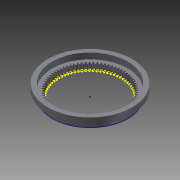
# Autodesk Inventor part: Stirnzahnrad1
Saved by Autodesk Inventor 2014 (Build 180170000, 170)
## iProperties
Created: 2013-05-23
Part Number: Stirnzahnrad1
Material: Steel
Document SubType Name: Modeling
Designer: hartmann
Categories: <?xml version="1.0" encoding="UTF-16"?> <MemberInstance><Categories><FamilyTemplate><FamilyTemplateParameter ValueType="xs:double" Id="1" ObjectReferenceKey="da_z" ObjectType="kUserParameterObject"/><FamilyTemplateParameter ValueType="xs:double" Id="2" ObjectReferenceKey="da_b" ObjectType="kUserParameterObject"/><FamilyTemplateParameter ValueType="xs:double" Id="3" ObjectReferenceKey="da_beta" ObjectType="kUserParameterObject"/><FamilyTemplateParameter ValueType="xs:double" Id="4" ObjectReferenceKey="da_da" ObjectType="kUserParameterObject"/><FamilyTemplateParameter ValueType="xs:double" Id="5" ObjectReferenceKey="da_aw" ObjectType="kUserParameterObject"/><FamilyTemplateParameter ValueType="xs:string" Id="6" ObjectReferenceKey="EAIAABAAAACIAQAAAAAAAIAAAAAAAAAA" ObjectType="83910656" SubObjectId="SurfaceGeometry"/></FamilyTemplate><ParamToTemplateMap><ParamToTemplate CategoryParameter="//CategoryParameter[@InternalName='046C89C9-8512-4d59-83FE-43B91F4F132A']" TemplateParameter="1"/><ParamToTemplate CategoryParameter="//CategoryParameter[@InternalName='2552DF32-E462-4b46-AEBF-C6C7768E72AC']" TemplateParameter="2"/><ParamToTemplate CategoryParameter="//CategoryParameter[@InternalName='C9EE641D-15FC-4fae-A226-E94C4372FDD7']" TemplateParameter="3"/><ParamToTemplate><ParamToTemplate CategoryParameter="//CategoryParameter[@InternalName='00B6519A-459B-49c7-AD84-2E56D39A5744']" ConstantValue="0.000000"/></ParamToTemplate><ParamToTemplate><ParamToTemplate CategoryParameter="//CategoryParameter[@InternalName='04B31F0E-C7A6-4894-AA32-9629BEFACF47']" ConstantValue="1.000000"/></ParamToTemplate><ParamToTemplate><ParamToTemplate CategoryParameter="//CategoryParameter[@InternalName='43CBEC2E-7847-49e7-A936-2F7889FCB2D9']" ConstantValue="0.250000"/></ParamToTemplate><ParamToTemplate><ParamToTemplate CategoryParameter="//CategoryParameter[@InternalName='B1EFC894-105D-4ebd-86BF-FA20ED196853']" ConstantValue="0.350000"/></ParamToTemplate><ParamToTemplate><ParamToTemplate CategoryParameter="//CategoryParameter[@InternalName='51175063-3D10-4879-93E8-6246FE8B403D']" ConstantValue="2060000000.000000"/></ParamToTemplate><ParamToTemplate><ParamToTemplate CategoryParameter="//CategoryParameter[@InternalName='A3A52E27-4454-46a9-B0BD-C932399B70AF']" ConstantValue="0.300000"/></ParamToTemplate><ParamToTemplate><ParamToTemplate CategoryParameter="//CategoryParameter[@InternalName='91B76062-C214-41d9-B1B9-14D2AB99603D']" ConstantValue="0.030000"/></ParamToTemplate><ParamToTemplate><ParamToTemplate CategoryParameter="//CategoryParameter[@InternalName='374E806E-8B8A-4dda-A9AA-1039D6500AD2']" ConstantValue="33.333333"/></ParamToTemplate><ParamToTemplate><ParamToTemplate CategoryParameter="//CategoryParameter[@InternalName='2D373A89-B862-43d6-8D0B-0CBF12AB9F6C']" ConstantValue="0.349066"/></ParamToTemplate><ParamToTemplate CategoryParameter="//CategoryParameter[@InternalName='37777632-D6A2-4fac-9D53-DB8ACD95C989']" TemplateParameter="4"/><ParamToTemplate CategoryParameter="//CategoryParameter[@InternalName='FD1017F1-B727-4f7e-9707-0F86F1FF9423']" TemplateParameter="5"/><ParamToTemplate><ParamToTemplate CategoryParameter="//CategoryParameter[@InternalName='9E1B4470-B2D3-4ff1-B813-535BB4CDF51A']" ConstantValue="3520000.000000"/></ParamToTemplate><ParamToTemplate><ParamToTemplate CategoryParameter="//CategoryParameter[@InternalName='F8452263-BFF6-458c-9FB1-07C4B99E95CD']" ConstantValue="11400000.000000"/></ParamToTemplate><ParamToTemplate><ParamToTemplate CategoryParameter="//CategoryParameter[@InternalName='3E3BB259-FD49-497f-8171-6EBC954A3479']" ConstantValue="2.000000"/></ParamToTemplate><ParamToTemplate CategoryParameter="//CategoryParameter[@InternalName='27C3BAF2-7550-4e4b-AE2C-0DB134B7D9B7']" TemplateParameter="6"/></ParamToTemplateMap><Category DisplayName="Gear" InternalName="DC85795E-93AB-48d5-8EEE-5A27447B64BD" Mnemonic="Gear"><CategoryParameter DisplayName="z" InternalName="046C89C9-8512-4d59-83FE-43B91F4F132A" Mnemonic="z"/><CategoryParameter DisplayName="b" InternalName="2552DF32-E462-4b46-AEBF-C6C7768E72AC" Mnemonic="b"/><CategoryParameter DisplayName="||b|" InternalName="C9EE641D-15FC-4fae-A226-E94C4372FDD7" Mnemonic="beta"/><CategoryParameter DisplayName="x" InternalName="00B6519A-459B-49c7-AD84-2E56D39A5744" Mnemonic="x"/><CategoryParameter DisplayName="a*" InternalName="04B31F0E-C7A6-4894-AA32-9629BEFACF47" Mnemonic="a"/><CategoryParameter DisplayName="c*" InternalName="43CBEC2E-7847-49e7-A936-2F7889FCB2D9" Mnemonic="c"/><CategoryParameter DisplayName="r|.f|*" InternalName="B1EFC894-105D-4ebd-86BF-FA20ED196853" Mnemonic="rf"/><CategoryParameter DisplayName="E" InternalName="51175063-3D10-4879-93E8-6246FE8B403D" Mnemonic="E"/><CategoryParameter DisplayName="||m|" InternalName="A3A52E27-4454-46a9-B0BD-C932399B70AF" Mnemonic="mi"/><Category DisplayName="SpurGear" InternalName="26C5A22E-A91E-4dfd-A3B3-23CCAFAE1764" Mnemonic="SpurGear"><CategoryParameter DisplayName="m" InternalName="91B76062-C214-41d9-B1B9-14D2AB99603D" Mnemonic="m"/><CategoryParameter DisplayName="P" InternalName="374E806E-8B8A-4dda-A9AA-1039D6500AD2" Mnemonic="PP"/><CategoryParameter DisplayName="||a|" InternalName="2D373A89-B862-43d6-8D0B-0CBF12AB9F6C" Mnemonic="alpha"/><CategoryParameter DisplayName="d|.a|" InternalName="37777632-D6A2-4fac-9D53-DB8ACD95C989" Mnemonic="da"/><CategoryParameter DisplayName="a|.w|" InternalName="FD1017F1-B727-4f7e-9707-0F86F1FF9423" Mnemonic="aw"/><CategoryParameter DisplayName="||s||.Flim|" InternalName="9E1B4470-B2D3-4ff1-B813-535BB4CDF51A" Mnemonic="sFlim"/><CategoryParameter DisplayName="||s||.Hlim|" InternalName="F8452263-BFF6-458c-9FB1-07C4B99E95CD" Mnemonic="sHlim"/><CategoryParameter DisplayName="Typ" InternalName="3E3BB259-FD49-497f-8171-6EBC954A3479" Mnemonic="type"/><Category DisplayName="InternalSpurGear" InternalName="7CF704F6-14A9-42f8-93CE-E71DF57C2B55" Mnemonic="InternalSpurGear"><CategoryParameter DisplayName="PitchDiameter" InternalName="27C3BAF2-7550-4e4b-AE2C-0DB134B7D9B7" Mnemonic="IDS_PITCHDIAM"/></Category></Category></Category></Categories></MemberInstance>
Density: 1 g/cm^3
Appearance: Steel
CustomPartVersion: 1
Author: hartmann
Autodesk Inventor part; units mm, degrees
sketch "Sketch1" plane through (0, 0, 0) normal (0, 0, 1) x (1, 0, 0)
  circle A0 centre (0, 0) radius 12.7875
  dimension "d0" = 25.575
  constraints: 1 centre point
  measures "d0" diameter of A0
extrude "Extrusion1" add sketch "Sketch1" along normal blind 2
ref_plane "Work Plane2" through (0, 0, 1) normal (0, 0, 1) x (1, 0, 0)
sketch "Sketch2" plane through (0, 0, 0) normal (0, 0, -1) x (-1, 0, 0)
  circle A0 centre (0, 0) radius 12.7875 projected
  circle A1 centre (0, 0) radius 11.25
  dimension "d3" = 22.5
  constraints: 1 centre point, 1 coincident
  measures "d3" diameter of A1
surface extrude "Flankendurchmesser" sketch "Sketch2" against normal through all shown no curves A1
ref_plane "Work Plane8" through (0, 0, 0) normal (0.9991228, 0.0418757, 0) x (0, 0, 1)
ref_plane "Work Plane9" through (0, 0, 0) normal (1, 0, 0) x (0, 1, 0)
spur gear teeth "Stirnzahnrad" teeth 75 pitch diameter 22.5 tip diameter 21.9 root diameter 23.25 face width 2 start plane through (0, 0, 0) normal (0, 0, -1) x (-1, 0, 0)
sketch "Skizze4" plane through (0, 0, 2) normal (0, 0, 1) x (1, 0, 0)
  circle A0 centre (0, 0) radius 12.7875 projected
  circle A1 centre (0, 0) radius 14.2875
  arc A2 (1.2586, -10.8774) -> (1.4861, -10.8487) centre (0, 0) ccw projected
  circle A3 centre (0, 0) radius 14.2875
  dimension "d53" = 1.5
  constraints: 2 centre point, 2 coincident, 1 concentric
  measures "d53" radial gap between concentric circles of A0 A1
extrude "Extrusion2" add sketch "Skizze4" along normal blind 2
sketch "Skizze6" plane through (0, 0, 0) normal (0, 0, -1) x (-1, 0, 0)
  arc A0 (-1.2586, -10.8774) -> (-1.094, -11.5734) centre (2.6832, -10.3129) ccw projected
  arc A1 (-1.4861, -10.8487) -> (-1.2586, -10.8774) centre (0, 0) ccw projected
  arc A2 (-1.8186, -11.4819) -> (-1.4861, -10.8487) centre (-5.1636, -9.3216) ccw projected
  arc A3 (-2.0586, -11.4413) -> (-1.8186, -11.4819) centre (0, 0) ccw projected
  arc A4 (-2.1643, -10.734) -> (-2.0586, -11.4413) centre (1.8108, -10.5013) ccw projected
  arc A5 (-2.3887, -10.6863) -> (-2.1643, -10.734) centre (0, 0) ccw projected
  arc A6 (-2.773, -11.2894) -> (-2.3887, -10.6863) centre (-5.9255, -8.8569) ccw projected
  arc A7 (-3.0088, -11.2289) -> (-2.773, -11.2894) centre (0, 0) ccw projected
  arc A8 (-3.055, -10.5152) -> (-3.0088, -11.2289) centre (0.9257, -10.616) ccw projected
  arc A9 (-3.2745, -10.4489) -> (-3.055, -10.5152) centre (0, 0) ccw projected
  arc A10 (-3.7079, -11.0178) -> (-3.2745, -10.4489) centre (-6.6458, -8.33) ccw projected
  arc A11 (-3.9378, -10.9377) -> (-3.7079, -11.0178) centre (0, 0) ccw projected
  arc A12 (-3.9241, -10.2227) -> (-3.9378, -10.9377) centre (0.0342, -10.6562) ccw projected
  arc A13 (-4.1374, -10.1383) -> (-3.9241, -10.2227) centre (0, 0) ccw projected
  arc A14 (-4.6168, -10.6689) -> (-4.1374, -10.1383) centre (-7.3196, -7.7446) ccw projected
  arc A15 (-4.8393, -10.5699) -> (-4.6168, -10.6689) centre (0, 0) ccw projected
  arc A16 (-4.7658, -9.8585) -> (-4.8393, -10.5699) centre (-0.8576, -10.6217) ccw projected
  arc A17 (-4.9712, -9.7565) -> (-4.7658, -9.8585) centre (0, 0) ccw projected
  arc A18 (-5.4934, -10.2452) -> (-4.9712, -9.7565) centre (-7.942, -7.105) ccw projected
  arc A19 (-5.7068, -10.1279) -> (-5.4934, -10.2452) centre (0, 0) ccw projected
  arc A20 (-5.574, -9.4251) -> (-5.7068, -10.1279) centre (-1.7434, -10.5127) ccw projected
  arc A21 (-5.7702, -9.3063) -> (-5.574, -9.4251) centre (0, 0) ccw projected
  arc A22 (-6.3314, -9.7495) -> (-5.7702, -9.3063) centre (-8.5086, -6.4155) ccw projected
  arc A23 (-6.5342, -9.6148) -> (-6.3314, -9.7495) centre (0, 0) ccw projected
  arc A24 (-6.3431, -8.9256) -> (-6.5342, -9.6148) centre (-2.617, -10.3299) ccw projected
  arc A25 (-6.5287, -8.7909) -> (-6.3431, -8.9256) centre (0, 0) ccw projected
  arc A26 (-7.125, -9.1856) -> (-6.5287, -8.7909) centre (-9.0156, -5.681) ccw projected
  arc A27 (-7.3158, -9.0343) -> (-7.125, -9.1856) centre (0, 0) ccw projected
  arc A28 (-7.0678, -8.3636) -> (-7.3158, -9.0343) centre (-3.4722, -10.0747) ccw projected
  arc A29 (-7.2414, -8.2137) -> (-7.0678, -8.3636) centre (0, 0) ccw projected
  arc A30 (-7.8687, -8.5571) -> (-7.2414, -8.2137) centre (-9.4594, -4.9067) ccw projected
  arc A31 (-8.0462, -8.3905) -> (-7.8687, -8.5571) centre (0, 0) ccw projected
  arc A32 (-7.7428, -7.7428) -> (-8.0462, -8.3905) centre (-4.3031, -9.7488) ccw projected
  arc A33 (-7.9033, -7.579) -> (-7.7428, -7.7428) centre (0, 0) ccw projected
  arc A34 (-8.5571, -7.8687) -> (-7.9033, -7.579) centre (-9.8368, -4.0979) ccw projected
  arc A35 (-8.72, -7.6878) -> (-8.5571, -7.8687) centre (0, 0) ccw projected
  arc A36 (-8.3636, -7.0678) -> (-8.72, -7.6878) centre (-5.1037, -9.3545) ccw projected
  arc A37 (-8.5097, -6.8911) -> (-8.3636, -7.0678) centre (0, 0) ccw projected
  arc A38 (-9.1856, -7.125) -> (-8.5097, -6.8911) centre (-10.1452, -3.2605) ccw projected
  arc A39 (-9.3328, -6.9311) -> (-9.1856, -7.125) centre (0, 0) ccw projected
  arc A40 (-8.9256, -6.3431) -> (-9.3328, -6.9311) centre (-5.8686, -8.8947) ccw projected
  arc A41 (-9.0565, -6.1548) -> (-8.9256, -6.3431) centre (0, 0) ccw projected
  arc A42 (-9.7495, -6.3314) -> (-9.0565, -6.1548) centre (-10.3824, -2.4001) ccw projected
  arc A43 (-9.88, -6.1259) -> (-9.7495, -6.3314) centre (0, 0) ccw projected
  arc A44 (-9.4251, -5.574) -> (-9.88, -6.1259) centre (-6.5923, -8.3724) ccw projected
  arc A45 (-9.5398, -5.3754) -> (-9.4251, -5.574) centre (0, 0) ccw projected
  arc A46 (-10.2452, -5.4934) -> (-9.5398, -5.3754) centre (-10.5469, -1.5229) ccw projected
  arc A47 (-10.358, -5.2776) -> (-10.2452, -5.4934) centre (0, 0) ccw projected
  arc A48 (-9.8585, -4.7658) -> (-10.358, -5.2776) centre (-7.2698, -7.7914) ccw projected
  arc A49 (-9.9561, -4.5583) -> (-9.8585, -4.7658) centre (0, 0) ccw projected
  arc A50 (-10.6689, -4.6168) -> (-9.9561, -4.5583) centre (-10.6373, -0.635) ccw projected
  arc A51 (-10.7632, -4.3924) -> (-10.6689, -4.6168) centre (0, 0) ccw projected
  arc A52 (-10.2227, -3.9241) -> (-10.7632, -4.3924) centre (-7.8962, -7.1558) ccw projected
  arc A53 (-10.3026, -3.7092) -> (-10.2227, -3.9241) centre (0, 0) ccw projected
  arc A54 (-11.0178, -3.7079) -> (-10.3026, -3.7092) centre (-10.6531, 0.2573) ccw projected
  arc A55 (-11.093, -3.4763) -> (-11.0178, -3.7079) centre (0, 0) ccw projected
  arc A56 (-10.5152, -3.055) -> (-11.093, -3.4763) centre (-8.4673, -6.4699) ccw projected
  arc A57 (-10.5769, -2.8341) -> (-10.5152, -3.055) centre (0, 0) ccw projected
  arc A58 (-11.2894, -2.773) -> (-10.5769, -2.8341) centre (-10.5942, 1.1479) ccw projected
  arc A59 (-11.345, -2.5359) -> (-11.2894, -2.773) centre (0, 0) ccw projected
  arc A60 (-10.734, -2.1643) -> (-11.345, -2.5359) centre (-8.979, -5.7387) ccw projected
  arc A61 (-10.7769, -1.9391) -> (-10.734, -2.1643) centre (0, 0) ccw projected
  arc A62 (-11.4819, -1.8186) -> (-10.7769, -1.9391) centre (-10.461, 2.0303) ccw projected
  arc A63 (-11.5174, -1.5777) -> (-11.4819, -1.8186) centre (0, 0) ccw projected
  arc A64 (-10.8774, -1.2586) -> (-11.5174, -1.5777) centre (-9.4277, -4.9672) ccw projected
  arc A65 (-10.9014, -1.0305) -> (-10.8774, -1.2586) centre (0, 0) ccw projected
  arc A66 (-11.5938, -0.8514) -> (-10.9014, -1.0305) centre (-10.2545, 2.8986) ccw projected
  arc A67 (-11.6091, -0.6084) -> (-11.5938, -0.8514) centre (0, 0) ccw projected
  arc A68 (-10.9446, -0.3439) -> (-11.6091, -0.6084) centre (-9.8103, -4.1609) ccw projected
  arc A69 (-10.9494, -0.1147) -> (-10.9446, -0.3439) centre (0, 0) ccw projected
  arc A70 (-11.6244, 0.1217) -> (-10.9494, -0.1147) centre (-9.9759, 3.7465) ccw projected
  arc A71 (-11.6193, 0.3652) -> (-11.6244, 0.1217) centre (0, 0) ccw projected
  arc A72 (-10.935, 0.5731) -> (-11.6193, 0.3652) centre (-10.1241, -3.3254) ccw projected
  arc A73 (-10.9206, 0.802) -> (-10.935, 0.5731) centre (0, 0) ccw projected
  arc A74 (-11.5734, 1.094) -> (-10.9206, 0.802) centre (-9.6275, 4.5681) ccw projected
  arc A75 (-11.548, 1.3361) -> (-11.5734, 1.094) centre (0, 0) ccw projected
  arc A76 (-10.8487, 1.4861) -> (-11.548, 1.3361) centre (-10.3668, -2.4666) ccw projected
  arc A77 (-10.8152, 1.713) -> (-10.8487, 1.4861) centre (0, 0) ccw projected
  arc A78 (-11.4413, 2.0586) -> (-10.8152, 1.713) centre (-9.2114, 5.3577) ccw projected
  arc A79 (-11.3957, 2.2978) -> (-11.4413, 2.0586) centre (0, 0) ccw projected
  arc A80 (-10.6863, 2.3887) -> (-11.3957, 2.2978) centre (-10.5369, -1.5905) ccw projected
  arc A81 (-10.6339, 2.6119) -> (-10.6863, 2.3887) centre (0, 0) ccw projected
  arc A82 (-11.2289, 3.0088) -> (-10.6339, 2.6119) centre (-8.7308, 6.1097) ccw projected
  arc A83 (-11.1634, 3.2433) -> (-11.2289, 3.0088) centre (0, 0) ccw projected
  arc A84 (-10.4489, 3.2745) -> (-11.1634, 3.2433) centre (-10.633, -0.7032) ccw projected
  arc A85 (-10.3781, 3.4926) -> (-10.4489, 3.2745) centre (0, 0) ccw projected
  arc A86 (-10.9377, 3.9378) -> (-10.3781, 3.4926) centre (-8.189, 6.8188) ccw projected
  arc A87 (-10.8529, 4.166) -> (-10.9377, 3.9378) centre (0, 0) ccw projected
  arc A88 (-10.1383, 4.1374) -> (-10.8529, 4.166) centre (-10.6546, 0.189) ccw projected
  arc A89 (-10.0494, 4.3488) -> (-10.1383, 4.1374) centre (0, 0) ccw projected
  arc A90 (-10.5699, 4.8393) -> (-10.0494, 4.3488) centre (-7.5897, 7.4802) ccw projected
  arc A91 (-10.4662, 5.0596) -> (-10.5699, 4.8393) centre (0, 0) ccw projected
  arc A92 (-9.7565, 4.9712) -> (-10.4662, 5.0596) centre (-10.6014, 1.0799) ccw projected
  arc A93 (-9.6503, 5.1744) -> (-9.7565, 4.9712) centre (0, 0) ccw projected
  arc A94 (-10.1279, 5.7068) -> (-9.6503, 5.1744) centre (-6.9371, 8.089) ccw projected
  arc A95 (-10.0061, 5.9176) -> (-10.1279, 5.7068) centre (0, 0) ccw projected
  arc A96 (-9.3063, 5.7702) -> (-10.0061, 5.9176) centre (-10.4738, 1.9632) ccw projected
  arc A97 (-9.1834, 5.9638) -> (-9.3063, 5.7702) centre (0, 0) ccw projected
  arc A98 (-9.6148, 6.5342) -> (-9.1834, 5.9638) centre (-6.2359, 8.6411) ccw projected
  arc A99 (-9.4759, 6.7341) -> (-9.6148, 6.5342) centre (0, 0) ccw projected
  arc A100 (-8.7909, 6.5287) -> (-9.4759, 6.7341) centre (-10.2728, 2.8328) ccw projected
  arc A101 (-8.6522, 6.7113) -> (-8.7909, 6.5287) centre (0, 0) ccw projected
  arc A102 (-9.0343, 7.3158) -> (-8.6522, 6.7113) centre (-5.491, 9.1326) ccw projected
  arc A103 (-8.8791, 7.5034) -> (-9.0343, 7.3158) centre (0, 0) ccw projected
  arc A104 (-8.2137, 7.2414) -> (-8.8791, 7.5034) centre (-9.9998, 3.6824) ccw projected
  arc A105 (-8.0603, 7.4118) -> (-8.2137, 7.2414) centre (0, 0) ccw projected
  arc A106 (-8.3905, 8.0462) -> (-8.0603, 7.4118) centre (-4.7075, 9.5601) ccw projected
  arc A107 (-8.2201, 8.2201) -> (-8.3905, 8.0462) centre (0, 0) ccw projected
  arc A108 (-7.579, 7.9033) -> (-8.2201, 8.2201) centre (-9.6566, 4.5063) ccw projected
  arc A109 (-7.4118, 8.0603) -> (-7.579, 7.9033) centre (0, 0) ccw projected
  arc A110 (-7.6878, 8.72) -> (-7.4118, 8.0603) centre (-3.891, 9.9205) ccw projected
  arc A111 (-7.5034, 8.8791) -> (-7.6878, 8.72) centre (0, 0) ccw projected
  arc A112 (-6.8911, 8.5097) -> (-7.5034, 8.8791) centre (-9.2456, 5.2985) ccw projected
  arc A113 (-6.7113, 8.6522) -> (-6.8911, 8.5097) centre (0, 0) ccw projected
  arc A114 (-6.9311, 9.3328) -> (-6.7113, 8.6522) centre (-3.0473, 10.2113) ccw projected
  arc A115 (-6.7341, 9.4759) -> (-6.9311, 9.3328) centre (0, 0) ccw projected
  arc A116 (-6.1548, 9.0565) -> (-6.7341, 9.4759) centre (-8.7698, 6.0536) ccw projected
  arc A117 (-5.9638, 9.1834) -> (-6.1548, 9.0565) centre (0, 0) ccw projected
  arc A118 (-6.1259, 9.88) -> (-5.9638, 9.1834) centre (-2.1821, 10.4304) ccw projected
  arc A119 (-5.9176, 10.0061) -> (-6.1259, 9.88) centre (0, 0) ccw projected
  arc A120 (-5.3754, 9.5398) -> (-5.9176, 10.0061) centre (-8.2325, 6.7662) ccw projected
  arc A121 (-5.1744, 9.6503) -> (-5.3754, 9.5398) centre (0, 0) ccw projected
  arc A122 (-5.2776, 10.358) -> (-5.1744, 9.6503) centre (-1.3017, 10.5764) ccw projected
  arc A123 (-5.0596, 10.4662) -> (-5.2776, 10.358) centre (0, 0) ccw projected
  arc A124 (-4.5583, 9.9561) -> (-5.0596, 10.4662) centre (-7.6375, 7.4313) ccw projected
  arc A125 (-4.3488, 10.0494) -> (-4.5583, 9.9561) centre (0, 0) ccw projected
  arc A126 (-4.3924, 10.7632) -> (-4.3488, 10.0494) centre (-0.4121, 10.6483) ccw projected
  arc A127 (-4.166, 10.8529) -> (-4.3924, 10.7632) centre (0, 0) ccw projected
  arc A128 (-3.7092, 10.3026) -> (-4.166, 10.8529) centre (-6.9888, 8.0444) ccw projected
  arc A129 (-3.4926, 10.3781) -> (-3.7092, 10.3026) centre (0, 0) ccw projected
  arc A130 (-3.4763, 11.093) -> (-3.4926, 10.3781) centre (0.4804, 10.6454) ccw projected
  arc A131 (-3.2433, 11.1634) -> (-3.4763, 11.093) centre (0, 0) ccw projected
  arc A132 (-2.8341, 10.5769) -> (-3.2433, 11.1634) centre (-6.2912, 8.601) ccw projected
  arc A133 (-2.6119, 10.6339) -> (-2.8341, 10.5769) centre (0, 0) ccw projected
  arc A134 (-2.5359, 11.345) -> (-2.6119, 10.6339) centre (1.3695, 10.5679) ccw projected
  arc A135 (-2.2978, 11.3957) -> (-2.5359, 11.345) centre (0, 0) ccw projected
  arc A136 (-1.9391, 10.7769) -> (-2.2978, 11.3957) centre (-5.5494, 9.0972) ccw projected
  arc A137 (-1.713, 10.8152) -> (-1.9391, 10.7769) centre (0, 0) ccw projected
  arc A138 (-1.5777, 11.5174) -> (-1.713, 10.8152) centre (2.249, 10.4162) ccw projected
  arc A139 (-1.3361, 11.548) -> (-1.5777, 11.5174) centre (0, 0) ccw projected
  arc A140 (-1.0305, 10.9014) -> (-1.3361, 11.548) centre (-4.7687, 9.5297) ccw projected
  arc A141 (-0.802, 10.9206) -> (-1.0305, 10.9014) centre (0, 0) ccw projected
  arc A142 (-0.6084, 11.6091) -> (-0.802, 10.9206) centre (3.1127, 10.1915) ccw projected
  arc A143 (-0.3652, 11.6193) -> (-0.6084, 11.6091) centre (0, 0) ccw projected
  arc A144 (-0.1147, 10.9494) -> (-0.3652, 11.6193) centre (-3.9546, 9.8953) ccw projected
  arc A145 (0.1147, 10.9494) -> (-0.1147, 10.9494) centre (0, 0) ccw projected
  arc A146 (0.3652, 11.6193) -> (0.1147, 10.9494) centre (3.9546, 9.8953) ccw projected
  arc A147 (0.6084, 11.6091) -> (0.3652, 11.6193) centre (0, 0) ccw projected
  arc A148 (0.802, 10.9206) -> (0.6084, 11.6091) centre (-3.1127, 10.1915) ccw projected
  arc A149 (1.0305, 10.9014) -> (0.802, 10.9206) centre (0, 0) ccw projected
  arc A150 (1.3361, 11.548) -> (1.0305, 10.9014) centre (4.7687, 9.5297) ccw projected
  arc A151 (1.5777, 11.5174) -> (1.3361, 11.548) centre (0, 0) ccw projected
  arc A152 (1.713, 10.8152) -> (1.5777, 11.5174) centre (-2.249, 10.4162) ccw projected
  arc A153 (1.9391, 10.7769) -> (1.713, 10.8152) centre (0, 0) ccw projected
  arc A154 (2.2978, 11.3957) -> (1.9391, 10.7769) centre (5.5494, 9.0972) ccw projected
  arc A155 (2.5359, 11.345) -> (2.2978, 11.3957) centre (0, 0) ccw projected
  arc A156 (2.6119, 10.6339) -> (2.5359, 11.345) centre (-1.3695, 10.5679) ccw projected
  arc A157 (2.8341, 10.5769) -> (2.6119, 10.6339) centre (0, 0) ccw projected
  arc A158 (3.2433, 11.1634) -> (2.8341, 10.5769) centre (6.2912, 8.601) ccw projected
  arc A159 (3.4763, 11.093) -> (3.2433, 11.1634) centre (0, 0) ccw projected
  arc A160 (3.4926, 10.3781) -> (3.4763, 11.093) centre (-0.4804, 10.6454) ccw projected
  arc A161 (3.7092, 10.3026) -> (3.4926, 10.3781) centre (0, 0) ccw projected
  arc A162 (4.166, 10.8529) -> (3.7092, 10.3026) centre (6.9888, 8.0444) ccw projected
  arc A163 (4.3924, 10.7632) -> (4.166, 10.8529) centre (0, 0) ccw projected
  arc A164 (4.3488, 10.0494) -> (4.3924, 10.7632) centre (0.4121, 10.6483) ccw projected
  arc A165 (4.5583, 9.9561) -> (4.3488, 10.0494) centre (0, 0) ccw projected
  arc A166 (5.0596, 10.4662) -> (4.5583, 9.9561) centre (7.6375, 7.4313) ccw projected
  arc A167 (5.2776, 10.358) -> (5.0596, 10.4662) centre (0, 0) ccw projected
  arc A168 (5.1744, 9.6503) -> (5.2776, 10.358) centre (1.3017, 10.5764) ccw projected
  arc A169 (5.3754, 9.5398) -> (5.1744, 9.6503) centre (0, 0) ccw projected
  arc A170 (5.9176, 10.0061) -> (5.3754, 9.5398) centre (8.2325, 6.7662) ccw projected
  arc A171 (6.1259, 9.88) -> (5.9176, 10.0061) centre (0, 0) ccw projected
  arc A172 (5.9638, 9.1834) -> (6.1259, 9.88) centre (2.1821, 10.4304) ccw projected
  arc A173 (6.1548, 9.0565) -> (5.9638, 9.1834) centre (0, 0) ccw projected
  arc A174 (6.7341, 9.4759) -> (6.1548, 9.0565) centre (8.7698, 6.0536) ccw projected
  arc A175 (6.9311, 9.3328) -> (6.7341, 9.4759) centre (0, 0) ccw projected
  arc A176 (6.7113, 8.6522) -> (6.9311, 9.3328) centre (3.0473, 10.2113) ccw projected
  arc A177 (6.8911, 8.5097) -> (6.7113, 8.6522) centre (0, 0) ccw projected
  arc A178 (7.5034, 8.8791) -> (6.8911, 8.5097) centre (9.2456, 5.2985) ccw projected
  arc A179 (7.6878, 8.72) -> (7.5034, 8.8791) centre (0, 0) ccw projected
  arc A180 (7.4118, 8.0603) -> (7.6878, 8.72) centre (3.891, 9.9205) ccw projected
  arc A181 (7.579, 7.9033) -> (7.4118, 8.0603) centre (0, 0) ccw projected
  arc A182 (8.2201, 8.2201) -> (7.579, 7.9033) centre (9.6566, 4.5063) ccw projected
  arc A183 (8.3905, 8.0462) -> (8.2201, 8.2201) centre (0, 0) ccw projected
  arc A184 (8.0603, 7.4118) -> (8.3905, 8.0462) centre (4.7075, 9.5601) ccw projected
  arc A185 (8.2137, 7.2414) -> (8.0603, 7.4118) centre (0, 0) ccw projected
  arc A186 (8.8791, 7.5034) -> (8.2137, 7.2414) centre (9.9998, 3.6824) ccw projected
  arc A187 (9.0343, 7.3158) -> (8.8791, 7.5034) centre (0, 0) ccw projected
  arc A188 (8.6522, 6.7113) -> (9.0343, 7.3158) centre (5.491, 9.1326) ccw projected
  arc A189 (8.7909, 6.5287) -> (8.6522, 6.7113) centre (0, 0) ccw projected
  arc A190 (9.4759, 6.7341) -> (8.7909, 6.5287) centre (10.2728, 2.8328) ccw projected
  arc A191 (9.6148, 6.5342) -> (9.4759, 6.7341) centre (0, 0) ccw projected
  arc A192 (9.1834, 5.9638) -> (9.6148, 6.5342) centre (6.2359, 8.6411) ccw projected
  arc A193 (9.3063, 5.7702) -> (9.1834, 5.9638) centre (0, 0) ccw projected
  arc A194 (10.0061, 5.9176) -> (9.3063, 5.7702) centre (10.4738, 1.9632) ccw projected
  arc A195 (10.1279, 5.7068) -> (10.0061, 5.9176) centre (0, 0) ccw projected
  arc A196 (9.6503, 5.1744) -> (10.1279, 5.7068) centre (6.9371, 8.089) ccw projected
  arc A197 (9.7565, 4.9712) -> (9.6503, 5.1744) centre (0, 0) ccw projected
  arc A198 (10.4662, 5.0596) -> (9.7565, 4.9712) centre (10.6014, 1.0799) ccw projected
  arc A199 (10.5699, 4.8393) -> (10.4662, 5.0596) centre (0, 0) ccw projected
  arc A200 (10.0494, 4.3488) -> (10.5699, 4.8393) centre (7.5897, 7.4802) ccw projected
  arc A201 (10.1383, 4.1374) -> (10.0494, 4.3488) centre (0, 0) ccw projected
  arc A202 (10.8529, 4.166) -> (10.1383, 4.1374) centre (10.6546, 0.189) ccw projected
  arc A203 (10.9377, 3.9378) -> (10.8529, 4.166) centre (0, 0) ccw projected
  arc A204 (10.3781, 3.4926) -> (10.9377, 3.9378) centre (8.189, 6.8188) ccw projected
  arc A205 (10.4489, 3.2745) -> (10.3781, 3.4926) centre (0, 0) ccw projected
  arc A206 (11.1634, 3.2433) -> (10.4489, 3.2745) centre (10.633, -0.7032) ccw projected
  arc A207 (11.2289, 3.0088) -> (11.1634, 3.2433) centre (0, 0) ccw projected
  arc A208 (10.6339, 2.6119) -> (11.2289, 3.0088) centre (8.7308, 6.1097) ccw projected
  arc A209 (10.6863, 2.3887) -> (10.6339, 2.6119) centre (0, 0) ccw projected
  arc A210 (11.3957, 2.2978) -> (10.6863, 2.3887) centre (10.5369, -1.5905) ccw projected
  arc A211 (11.4413, 2.0586) -> (11.3957, 2.2978) centre (0, 0) ccw projected
  arc A212 (10.8152, 1.713) -> (11.4413, 2.0586) centre (9.2114, 5.3577) ccw projected
  arc A213 (10.8487, 1.4861) -> (10.8152, 1.713) centre (0, 0) ccw projected
  arc A214 (11.548, 1.3361) -> (10.8487, 1.4861) centre (10.3668, -2.4666) ccw projected
  arc A215 (11.5734, 1.094) -> (11.548, 1.3361) centre (0, 0) ccw projected
  arc A216 (10.9206, 0.802) -> (11.5734, 1.094) centre (9.6275, 4.5681) ccw projected
  arc A217 (10.935, 0.5731) -> (10.9206, 0.802) centre (0, 0) ccw projected
  arc A218 (11.6193, 0.3652) -> (10.935, 0.5731) centre (10.1241, -3.3254) ccw projected
  arc A219 (11.6244, 0.1217) -> (11.6193, 0.3652) centre (0, 0) ccw projected
  arc A220 (10.9494, -0.1147) -> (11.6244, 0.1217) centre (9.9759, 3.7465) ccw projected
  arc A221 (10.9446, -0.3439) -> (10.9494, -0.1147) centre (0, 0) ccw projected
  arc A222 (11.6091, -0.6084) -> (10.9446, -0.3439) centre (9.8103, -4.1609) ccw projected
  arc A223 (11.5938, -0.8514) -> (11.6091, -0.6084) centre (0, 0) ccw projected
  arc A224 (10.9014, -1.0305) -> (11.5938, -0.8514) centre (10.2545, 2.8986) ccw projected
  arc A225 (10.8774, -1.2586) -> (10.9014, -1.0305) centre (0, 0) ccw projected
  arc A226 (11.5174, -1.5777) -> (10.8774, -1.2586) centre (9.4277, -4.9672) ccw projected
  arc A227 (11.4819, -1.8186) -> (11.5174, -1.5777) centre (0, 0) ccw projected
  arc A228 (10.7769, -1.9391) -> (11.4819, -1.8186) centre (10.461, 2.0303) ccw projected
  arc A229 (10.734, -2.1643) -> (10.7769, -1.9391) centre (0, 0) ccw projected
  arc A230 (11.345, -2.5359) -> (10.734, -2.1643) centre (8.979, -5.7387) ccw projected
  arc A231 (11.2894, -2.773) -> (11.345, -2.5359) centre (0, 0) ccw projected
  arc A232 (10.5769, -2.8341) -> (11.2894, -2.773) centre (10.5942, 1.1479) ccw projected
  arc A233 (10.5152, -3.055) -> (10.5769, -2.8341) centre (0, 0) ccw projected
  arc A234 (11.093, -3.4763) -> (10.5152, -3.055) centre (8.4673, -6.4699) ccw projected
  arc A235 (11.0178, -3.7079) -> (11.093, -3.4763) centre (0, 0) ccw projected
  arc A236 (10.3026, -3.7092) -> (11.0178, -3.7079) centre (10.6531, 0.2573) ccw projected
  arc A237 (10.2227, -3.9241) -> (10.3026, -3.7092) centre (0, 0) ccw projected
  arc A238 (10.7632, -4.3924) -> (10.2227, -3.9241) centre (7.8962, -7.1558) ccw projected
  arc A239 (10.6689, -4.6168) -> (10.7632, -4.3924) centre (0, 0) ccw projected
  arc A240 (9.9561, -4.5583) -> (10.6689, -4.6168) centre (10.6373, -0.635) ccw projected
  arc A241 (9.8585, -4.7658) -> (9.9561, -4.5583) centre (0, 0) ccw projected
  arc A242 (10.358, -5.2776) -> (9.8585, -4.7658) centre (7.2698, -7.7914) ccw projected
  arc A243 (10.2452, -5.4934) -> (10.358, -5.2776) centre (0, 0) ccw projected
  arc A244 (9.5398, -5.3754) -> (10.2452, -5.4934) centre (10.5469, -1.5229) ccw projected
  arc A245 (9.4251, -5.574) -> (9.5398, -5.3754) centre (0, 0) ccw projected
  arc A246 (9.88, -6.1259) -> (9.4251, -5.574) centre (6.5923, -8.3724) ccw projected
  arc A247 (9.7495, -6.3314) -> (9.88, -6.1259) centre (0, 0) ccw projected
  arc A248 (9.0565, -6.1548) -> (9.7495, -6.3314) centre (10.3824, -2.4001) ccw projected
  arc A249 (8.9256, -6.3431) -> (9.0565, -6.1548) centre (0, 0) ccw projected
  arc A250 (9.3328, -6.9311) -> (8.9256, -6.3431) centre (5.8686, -8.8947) ccw projected
  arc A251 (9.1856, -7.125) -> (9.3328, -6.9311) centre (0, 0) ccw projected
  arc A252 (8.5097, -6.8911) -> (9.1856, -7.125) centre (10.1452, -3.2605) ccw projected
  arc A253 (8.3636, -7.0678) -> (8.5097, -6.8911) centre (0, 0) ccw projected
  arc A254 (8.72, -7.6878) -> (8.3636, -7.0678) centre (5.1037, -9.3545) ccw projected
  arc A255 (8.5571, -7.8687) -> (8.72, -7.6878) centre (0, 0) ccw projected
  arc A256 (7.9033, -7.579) -> (8.5571, -7.8687) centre (9.8368, -4.0979) ccw projected
  arc A257 (7.7428, -7.7428) -> (7.9033, -7.579) centre (0, 0) ccw projected
  arc A258 (8.0462, -8.3905) -> (7.7428, -7.7428) centre (4.3031, -9.7488) ccw projected
  arc A259 (7.8687, -8.5571) -> (8.0462, -8.3905) centre (0, 0) ccw projected
  arc A260 (7.2414, -8.2137) -> (7.8687, -8.5571) centre (9.4594, -4.9067) ccw projected
  arc A261 (7.0678, -8.3636) -> (7.2414, -8.2137) centre (0, 0) ccw projected
  arc A262 (7.3158, -9.0343) -> (7.0678, -8.3636) centre (3.4722, -10.0747) ccw projected
  arc A263 (7.125, -9.1856) -> (7.3158, -9.0343) centre (0, 0) ccw projected
  arc A264 (6.5287, -8.7909) -> (7.125, -9.1856) centre (9.0156, -5.681) ccw projected
  arc A265 (6.3431, -8.9256) -> (6.5287, -8.7909) centre (0, 0) ccw projected
  arc A266 (6.5342, -9.6148) -> (6.3431, -8.9256) centre (2.617, -10.3299) ccw projected
  arc A267 (6.3314, -9.7495) -> (6.5342, -9.6148) centre (0, 0) ccw projected
  arc A268 (5.7702, -9.3063) -> (6.3314, -9.7495) centre (8.5086, -6.4155) ccw projected
  arc A269 (5.574, -9.4251) -> (5.7702, -9.3063) centre (0, 0) ccw projected
  arc A270 (5.7068, -10.1279) -> (5.574, -9.4251) centre (1.7434, -10.5127) ccw projected
  arc A271 (5.4934, -10.2452) -> (5.7068, -10.1279) centre (0, 0) ccw projected
  arc A272 (4.9712, -9.7565) -> (5.4934, -10.2452) centre (7.942, -7.105) ccw projected
  arc A273 (4.7658, -9.8585) -> (4.9712, -9.7565) centre (0, 0) ccw projected
  arc A274 (4.8393, -10.5699) -> (4.7658, -9.8585) centre (0.8576, -10.6217) ccw projected
  arc A275 (4.6168, -10.6689) -> (4.8393, -10.5699) centre (0, 0) ccw projected
  arc A276 (4.1374, -10.1383) -> (4.6168, -10.6689) centre (7.3196, -7.7446) ccw projected
  arc A277 (3.9241, -10.2227) -> (4.1374, -10.1383) centre (0, 0) ccw projected
  arc A278 (3.9378, -10.9377) -> (3.9241, -10.2227) centre (-0.0342, -10.6562) ccw projected
  arc A279 (3.7079, -11.0178) -> (3.9378, -10.9377) centre (0, 0) ccw projected
  arc A280 (3.2745, -10.4489) -> (3.7079, -11.0178) centre (6.6458, -8.33) ccw projected
  arc A281 (3.055, -10.5152) -> (3.2745, -10.4489) centre (0, 0) ccw projected
  arc A282 (3.0088, -11.2289) -> (3.055, -10.5152) centre (-0.9257, -10.616) ccw projected
  arc A283 (2.773, -11.2894) -> (3.0088, -11.2289) centre (0, 0) ccw projected
  arc A284 (2.3887, -10.6863) -> (2.773, -11.2894) centre (5.9255, -8.8569) ccw projected
  arc A285 (2.1643, -10.734) -> (2.3887, -10.6863) centre (0, 0) ccw projected
  arc A286 (2.0586, -11.4413) -> (2.1643, -10.734) centre (-1.8108, -10.5013) ccw projected
  arc A287 (1.8186, -11.4819) -> (2.0586, -11.4413) centre (0, 0) ccw projected
  arc A288 (1.4861, -10.8487) -> (1.8186, -11.4819) centre (5.1636, -9.3216) ccw projected
  arc A289 (1.2586, -10.8774) -> (1.4861, -10.8487) centre (0, 0) ccw projected
  arc A290 (1.094, -11.5734) -> (1.2586, -10.8774) centre (-2.6832, -10.3129) ccw projected
  arc A291 (0.8514, -11.5938) -> (1.094, -11.5734) centre (0, 0) ccw projected
  arc A292 (0.5731, -10.935) -> (0.8514, -11.5938) centre (4.3655, -9.721) ccw projected
  arc A293 (0.3439, -10.9446) -> (0.5731, -10.935) centre (0, 0) ccw projected
  arc A294 (0.1217, -11.6244) -> (0.3439, -10.9446) centre (-3.5367, -10.0522) ccw projected
  arc A295 (-0.1217, -11.6244) -> (0.1217, -11.6244) centre (0, 0) ccw projected
  arc A296 (-0.3439, -10.9446) -> (-0.1217, -11.6244) centre (3.5367, -10.0522) ccw projected
  arc A297 (-0.5731, -10.935) -> (-0.3439, -10.9446) centre (0, 0) ccw projected
  arc A298 (-0.8514, -11.5938) -> (-0.5731, -10.935) centre (-4.3655, -9.721) ccw projected
  arc A299 (-1.094, -11.5734) -> (-0.8514, -11.5938) centre (0, 0) ccw projected
  circle A300 centre (0, 0) radius 12.7875 projected
  circle A301 centre (0, 0) radius 12.7875
  constraints: 1 centre point, 1 coincident, 1 concentric
equation "\"d0\" = 1.1 * da_df"
equation "\"d1\" = da_b"
equation "\"d3\" = da_dw"
equation "\"d16\" = da_aw"
equation "\"d47\" = da_aw"
equation "\"d52\" = da_aw"
equation "\"da_df\" = 23.25"
equation "\"da_b\" = 2"
equation "\"da_dw\" = 22.5"
equation "\"da_aw\" = 6.75"
body "Solid1"
body "Srf1"
